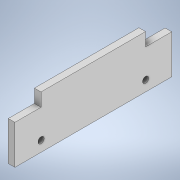
# Autodesk Inventor part: SideV1
Saved by Autodesk Inventor 2020 (Build 240168000, 168)
## iProperties
Created: 2020-06-07
Part Number: SideV1
Material: Generic
Document SubType Name: Modeling
Designer: Kitte_x
Density: 1 g/cm^3
Appearance: Default
Author: Kitte_x
Autodesk Inventor part; units mm, degrees
ref_plane "YZ Plane" through (0, 0, 0) normal (1, 0, 0) x (0, 1, 0)
ref_plane "XZ Plane" through (0, 0, 0) normal (0, 1, 0) x (-1, 0, 0)
ref_plane "XY Plane" through (0, 0, 0) normal (0, 0, 1) x (1, 0, 0)
sketch "Sketch1" plane through (0, 0, 0) normal (1, 0, 0) x (0, 1, 0)
  line L0 (-25, 75) -> (-25, -75)
  line L1 (-25, -75) -> (12.3, -75)
  line L2 (25, -50) -> (25, 50)
  line L3 (12.3, 75) -> (-25, 75)
  line L4 (12.3, 75) -> (12.3, 50)
  line L5 (12.3, 50) -> (25, 50)
  line L6 (12.3, -75) -> (12.3, -50)
  line L7 (12.3, -50) -> (25, -50)
  circle A0 centre (-15, 50) radius 2.95
  circle A1 centre (-15, -50) radius 2.95
  point P0 (0, 0)
  point P1 (25, 0)
  point P2 (0, 75)
  point P3 (18.65, 50)
  point P4 (18.65, -50)
  point P5 (25, 0)
  dimension "d0" = 150
  dimension "d2" = 12.7
  dimension "d3" = 25
  dimension "d4" = 12.7
  dimension "d5" = 25
  dimension "d6" = 50
  dimension "d7" = 5.9
  dimension "d8" = 5.9
  dimension "d9" = 10
  constraints: 16 end point, 5 perpendicular, 4 horizontal alignment, 4 midpoint, 3 vertical, 2 centre point, 2 vertical alignment, 1 point on line
  measures "d0" distance of L0.start L0.end
  measures "d2" distance between parallel lines of L2 L4
  measures "d3" distance between parallel lines of L3 L5
  measures "d4" distance between parallel lines of L2 L6
  measures "d5" distance between parallel lines of L1 L7
  measures "d6" distance between parallel lines of L0 L2
  measures "d7" diameter of A0
  measures "d8" diameter of A1
  measures "d9" distance from line of L0 A0.centre
extrude "Extrusion1" add sketch "Sketch1" along normal blind 6.35
body "Solid1"
